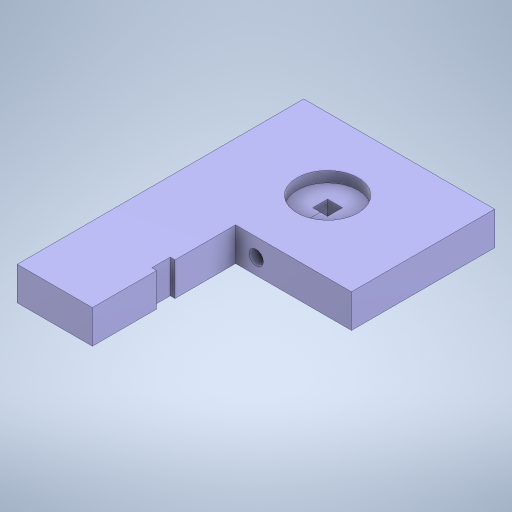
# Autodesk Inventor part: torch_light_injection_3d_pirnt_v0-1_20feb25
Saved by Autodesk Inventor 2024 (Build 280153000, 153)
## iProperties
Created: 2025-02-20
Part Number: torch_light_injection_3d_pirnt_v0-1_20feb25
Material: ABS Plastic
Document SubType Name: Modeling
Designer: phdgc
Density: 1.06 g/cm^3
Appearance: Smooth - White
Author: phdgc
Autodesk Inventor part; units mm, degrees
ref_plane "YZ Plane" through (0, 0, 0) normal (1, 0, 0) x (0, 1, 0)
ref_plane "XZ Plane" through (0, 0, 0) normal (0, 1, 0) x (-1, 0, 0)
ref_plane "XY Plane" through (0, 0, 0) normal (0, 0, 1) x (1, 0, 0)
sketch "Sketch1" plane through (0, 0, 0) normal (0, 1, 0) x (-1, 0, 0)
  line L0 (0, 0) -> (40, 0)
  line L1 (40, 0) -> (40, -60)
  line L2 (40, -60) -> (0, -60)
  line L3 (0, -60) -> (0, 0)
  dimension "d0" = 40
  dimension "d1" = 60
  constraints: 8 end point, 2 parallel, 1 horizontal, 1 perpendicular
  measures "d0" distance of L1.end L2.end
  measures "d1" distance of L0.end L1.end
extrude "Extrusion1" add sketch "Sketch1" along normal blind 7
sketch "Sketch2" plane through (0, 7, 0) normal (0, 1, 0) x (1, 0, 0)
  line L0 (-40, 0) -> (0, 0) projected
  line L1 (0, 0) -> (-24.276, 0)
  line L2 (-24.276, 0) -> (-24.276, 30)
  line L3 (-24.276, 30) -> (0, 30)
  line L4 (0, 30) -> (0, 0)
  dimension "d4" = 24.276
  dimension "d5" = 30
  constraints: 8 end point, 2 parallel, 1 horizontal, 1 perpendicular
  measures "d4" distance of L2.end L3.end
  measures "d5" distance of L1.end L2.end
extrude "Extrusion2" cut sketch "Sketch2" against normal through all
sketch "Sketch3" plane through (0, 7, 0) normal (0, 1, 0) x (1, 0, 0)
  circle A0 centre (-20, 45) radius 6.4
  point P0 (0, 0)
  dimension "d8" = 12.8
  constraints: 1 centre point
  measures "d8" diameter of A0
extrude "Extrusion3" cut sketch "Sketch3" against normal blind 2.25
sketch "Sketch4" plane through (-20, 4.75, -45) normal (0, 1, 0) x (1, 0, 0)
  line L0 (-1.55, -1.55) -> (1.55, -1.55)
  line L1 (1.55, -1.55) -> (1.55, 1.55)
  line L2 (1.55, 1.55) -> (-1.55, 1.55)
  line L3 (-1.55, 1.55) -> (-1.55, -1.55)
  line L4 (-1.55, -1.55) -> (1.55, 1.55) construction
  line L5 (1.55, -1.55) -> (-1.55, 1.55) construction
  point P0 (20, -45)
  point P1 (0, 0)
  dimension "d11" = 3.1
  dimension "d12" = 3.1
  constraints: 12 end point, 2 midpoint, 2 parallel, 1 horizontal, 1 perpendicular
  measures "d11" distance of L2.end L1.end
  measures "d12" distance of L1.end L0.end
extrude "Extrusion4" cut sketch "Sketch4" against normal blind 3
sketch "Sketch6" plane through (-18.45, 4.75, -43.45) normal (0, 0, -1) x (-1, 0, 0)
  circle A0 centre (1.5, -1.5) radius 1.5
  point P0 (-18.45, -4.75)
  dimension "d18" = 3
  constraints: 1 centre point
  measures "d18" diameter of A0
extrude "Extrusion6" cut sketch "Sketch6" against normal through all
sketch "Sketch7" plane through (0, 7, 0) normal (0, 1, 0) x (1, 0, 0)
  line L0 (-25.276, 17.3) -> (-21.276, 17.3)
  line L1 (-21.276, 17.3) -> (-21.276, 13.45)
  line L2 (-21.276, 13.45) -> (-25.276, 13.45)
  line L3 (-25.276, 13.45) -> (-25.276, 17.3)
  line L4 (-24.276, 0) -> (-24.276, 30) projected
  line L5 (-24.276, 30) -> (0, 30) projected
  point P0 (0, 0)
  dimension "d21" = 3.85
  dimension "d22" = 1
  dimension "d23" = 4
  dimension "d24" = 12.7
  constraints: 8 end point, 2 parallel, 1 horizontal, 1 perpendicular
  measures "d21" distance of L0.end L1.end
  measures "d22" distance between parallel lines of L4 L3
  measures "d23" distance of L1.end L2.end
  measures "d24" distance between parallel lines of L0 L5
extrude "Extrusion7" cut sketch "Sketch7" against normal through all
body "Solid1"
